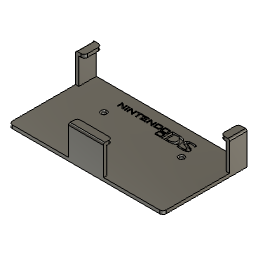
Nintendo DS Lite (Autodesk Fusion 360 design; units mm, degrees)
Autodesk Fusion 360 part; units mm, degrees
sketch "Sketch1" plane through (0, 0, 0) normal (0, 0, 1) x (1, 0, 0)
  line L0 (3, 0) -> (138, 0)
  line L1 (141, 3) -> (141, 77)
  line L2 (141, 77) -> (0, 77)
  line L3 (0, 77) -> (0, 3)
  line L4 (0, 77) -> (8, 77)
  line L5 (8, 77) -> (8, 61)
  line L6 (8, 61) -> (0, 61)
  line L7 (0, 61) -> (0, 77)
  line L8 (141, 77) -> (133, 77)
  line L9 (133, 77) -> (133, 64)
  line L10 (136, 61) -> (141, 61)
  line L11 (141, 61) -> (141, 77)
  line L12 (70.5, 77) -> (70.5, 0)
  line L13 (70.5, 0) -> (86.5, 0)
  line L14 (86.5, 0) -> (86.5, 5)
  line L15 (83.5, 8) -> (70.5, 8)
  line L16 (70.5, 8) -> (70.5, 0)
  line L17 (70.5, 0) -> (54.5, 0)
  line L18 (54.5, 0) -> (54.5, 5)
  line L19 (54.5, 8) -> (70.5, 8)
  line L20 (70.5, 8) -> (70.5, 0)
  line L21 (5, 61) -> (3, 61)
  line L22 (3, 61) -> (3, 77)
  line L23 (3, 77) -> (5, 77)
  line L24 (8, 74) -> (8, 64)
  line L25 (136, 77) -> (138, 77)
  line L26 (138, 77) -> (138, 61)
  line L27 (138, 61) -> (133, 61)
  line L28 (133, 61) -> (133, 74)
  line L29 (57.5, 8) -> (86.5, 8)
  line L30 (86.5, 8) -> (86.5, 3)
  line L31 (86.5, 3) -> (54.5, 3)
  line L32 (54.5, 3) -> (54.5, 8)
  arc A0 (8, 74) -> (5, 77) centre (5, 74) ccw
  arc A1 (136, 77) -> (133, 74) centre (136, 74) ccw
  arc A2 (133, 64) -> (136, 61) centre (136, 64) ccw
  arc A3 (5, 61) -> (8, 64) centre (5, 64) ccw
  arc A4 (57.5, 8) -> (54.5, 5) centre (57.5, 5) ccw
  arc A5 (86.5, 5) -> (83.5, 8) centre (83.5, 5) ccw
  arc A6 (0, 3) -> (3, 0) centre (3, 3) ccw
  arc A7 (138, 0) -> (141, 3) centre (138, 3) ccw
  point P0 (141, 0)
  dimension "d1" = 141
  dimension "d2" = 77
  dimension "d3" = 8
  dimension "d4" = 16
  dimension "d5" = 8
  dimension "d6" = 16
  dimension "d7" = 16
  dimension "d8" = 8
  dimension "d9" = 16
  dimension "d10" = 8
  dimension "d11" = 5
  dimension "d12" = 5
  dimension "d13" = 5
  dimension "d14" = 3
  dimension "d15" = 3
  dimension "d16" = 3
  dimension "d17" = 3
  constraint horizontal L0
  constraint vertical L1
  constraint horizontal L2
  constraint vertical L3
  constraint horizontal L4
  constraint vertical L5
  constraint horizontal L6
  constraint vertical L7
  constraint horizontal L8
  constraint vertical L9
  constraint horizontal L10
  constraint vertical L11
  constraint midpoint L2 L12.start
  constraint horizontal L13
  constraint vertical L14
  constraint horizontal L15
  constraint vertical L16
  constraint horizontal L17
  constraint vertical L18
  constraint horizontal L19
  constraint vertical L20
  constraint horizontal L21
  constraint vertical L22
  constraint horizontal L23
  constraint vertical L24
  constraint horizontal L25
  constraint vertical L26
  constraint horizontal L27
  constraint vertical L28
  constraint horizontal L29
  constraint vertical L30
  constraint horizontal L31
  constraint vertical L32
  constraint tangent L23 A0
  constraint tangent L24 A0
  constraint coincident L8.end L28
  constraint coincident L8.end L25
  constraint tangent L28 A1
  constraint tangent L25 A1
  constraint tangent L9 A2
  constraint tangent L10 A2
  constraint equal A1 A2
  constraint coincident L5.end L21
  constraint coincident L5.end L24
  constraint tangent L21 A3
  constraint tangent L24 A3
  constraint equal A1 A3
  constraint coincident L19.start L18
  constraint coincident L19.start L29
  constraint tangent L18 A4
  constraint tangent L29 A4
  constraint tangent L14 A5
  constraint tangent L15 A5
  constraint equal A4 A5
  constraint coincident L0 L12.end
  constraint coincident origin L0
  constraint coincident origin L3
  constraint tangent L0 A6
  constraint tangent L3 A6
  constraint coincident P0 L0
  constraint coincident P0 L1
  constraint tangent L0 A7
  constraint tangent L1 A7
  constraint equal A6 A7
  measures "d1" distance of origin P0
  measures "d2" distance of origin L2.end
  measures "d3" distance of L2.end L4.end
  measures "d4" distance of L2.end L6.end
  measures "d5" distance of L1.end L8.end
  measures "d6" distance of L1.end L10.end
  measures "d7" distance of L12.end L13.end
  measures "d8" distance of L12.end L15.end
  measures "d9" distance of L12.end L17.end
  measures "d10" distance of L12.end L15.end
  measures "d11" distance of L5.end L21.end
  measures "d12" distance of L8.end L25.end
  measures "d13" distance of L19.start L31.end
  measures "d14" radius of A0
  measures "d15" radius of A1
  measures "d16" radius of A4
  measures "d17" radius of A6
extrude "Extrude1" add sketch "Sketch1" along normal blind 30 contours L0 L12 L16 L17 L18 L20 L31 | L0 L12 L13 L14 L16 L20 L31 | L12 L16 L18 L19 L20 L29 L31 L32 A4 | L2 L3 L4 L6 L7 L22 | L12 L14 L15 L16 L20 L29 L30 L31 A5 | L2 L4 L5 L6 L21 L22 L23 L24 A0 A3 | L1 L2 L8 L10 L11 L26 | L2 L8 L9 L10 L25 L26 L27 L28 A1 A2 makes body 1 at (0, 71.6667, 10) makes body 2 at (141, 66.3333, 10) makes body 3 at (65.1667, 0, 10)
extrude "Extrude2" cut sketch "Sketch1" along normal blind 27 contours L12 L16 L18 L19 L20 L29 L31 L32 A4 | L12 L14 L15 L16 L20 L29 L30 L31 A5 | L2 L4 L5 L6 L21 L22 L23 L24 A0 A3 | L2 L8 L9 L10 L25 L26 L27 L28 A1 A2 bodies 1 2 3
extrude "Extrude3" add sketch "Sketch1" along normal blind 3 contours L0 L2 L3 L5 L6 L12 L18 L19 L21 L24 L29 L32 A6 | L12 L16 L18 L19 L20 L29 L31 L32 A4 | L0 L1 L2 L9 L10 L12 L14 L15 L27 L28 L29 L30 A7 | L12 L14 L15 L16 L20 L29 L30 L31 A5 | L19 L32 A4 | L2 L4 L5 L6 L21 L22 L23 L24 A0 A3 | L5 L6 A3 | L29 L30 A5 | L2 L4 L5 A0 | L2 L8 L9 A1 | L2 L8 L9 L10 L25 L26 L27 L28 A1 A2 | L27 L28 A2 bodies 1 2 3
fillet "Fillet1" radius 1.5 3 edges at (0, 69, 30) (70.5, 0, 30) (141, 69, 30) on bodies 1
sketch "Logo" plane through (0, 0, 3) normal (0, 0, 1) x (1, 0, 0)
  spline S0 degree 3 poles (75.8484, 66.8949) (75.8484, 67.0627) (75.8816, 67.0958) (76.0494, 67.0958) knots 0 0 0 0 1 1 1 1
  line L0 (76.0494, 67.0958) -> (79.7664, 67.0958)
  spline S1 degree 3 poles (79.7664, 67.0958) (79.9342, 67.0958) (79.9674, 67.0627) (79.9674, 66.8949) knots 2 2 2 2 3 3 3 3
  line L1 (79.9674, 66.8949) -> (79.9674, 64.2829)
  spline S2 degree 3 poles (79.9674, 64.2829) (79.9674, 64.1151) (79.9342, 64.082) (79.7664, 64.082) knots 4 4 4 4 5 5 5 5
  line L2 (79.7664, 64.082) -> (76.0494, 64.082)
  spline S3 degree 3 poles (76.0494, 64.082) (75.8816, 64.082) (75.8484, 64.1151) (75.8484, 64.2829) knots 6 6 6 6 7 7 7 7
  line L3 (75.8484, 64.2829) -> (75.8484, 66.8949)
  line L4 (75.0447, 66.9683) -> (75.0447, 64.2096)
  spline S4 degree 3 poles (75.0447, 64.2096) (75.0447, 63.6721) (75.4385, 63.2783) (75.976, 63.2783) knots 1 1 1 1 2 2 2 2
  line L5 (75.976, 63.2783) -> (79.8408, 63.2783)
  spline S5 degree 3 poles (79.8408, 63.2783) (80.3782, 63.2783) (80.7721, 63.6721) (80.7721, 64.2096) knots 3 3 3 3 4 4 4 4
  line L6 (80.7721, 64.2096) -> (80.7721, 66.9683)
  spline S6 degree 3 poles (80.7721, 66.9683) (80.7721, 67.5057) (80.3782, 67.8995) (79.8408, 67.8995) knots 5 5 5 5 6 6 6 6
  line L7 (79.8408, 67.8995) -> (75.976, 67.8995)
  spline S7 degree 3 poles (75.976, 67.8995) (75.4385, 67.8995) (75.0447, 67.5057) (75.0447, 66.9683) knots 7 7 7 7 8 8 8 8
  spline S8 degree 3 poles (75.8484, 61.6709) (75.8484, 61.8386) (75.8816, 61.8718) (76.0494, 61.8718) knots 0 0 0 0 1 1 1 1
  line L8 (76.0494, 61.8718) -> (79.7664, 61.8718)
  spline S9 degree 3 poles (79.7664, 61.8718) (79.9342, 61.8718) (79.9674, 61.8386) (79.9674, 61.6709) knots 2 2 2 2 3 3 3 3
  line L9 (79.9674, 61.6709) -> (79.9674, 59.0589)
  spline S10 degree 3 poles (79.9674, 59.0589) (79.9674, 58.8911) (79.9342, 58.8579) (79.7664, 58.8579) knots 4 4 4 4 5 5 5 5
  line L10 (79.7664, 58.8579) -> (76.0494, 58.8579)
  spline S11 degree 3 poles (76.0494, 58.8579) (75.8816, 58.8579) (75.8484, 58.8911) (75.8484, 59.0589) knots 6 6 6 6 7 7 7 7
  line L11 (75.8484, 59.0589) -> (75.8484, 61.6709)
  line L12 (75.0447, 61.7443) -> (75.0447, 58.9855)
  spline S12 degree 3 poles (75.0447, 58.9855) (75.0447, 58.4481) (75.4385, 58.0542) (75.976, 58.0542) knots 1 1 1 1 2 2 2 2
  line L13 (75.976, 58.0542) -> (79.8408, 58.0542)
  spline S13 degree 3 poles (79.8408, 58.0542) (80.3782, 58.0542) (80.7721, 58.4481) (80.7721, 58.9855) knots 3 3 3 3 4 4 4 4
  line L14 (80.7721, 58.9855) -> (80.7721, 61.7443)
  spline S14 degree 3 poles (80.7721, 61.7443) (80.7721, 62.2817) (80.3782, 62.6755) (79.8408, 62.6755) knots 5 5 5 5 6 6 6 6
  line L15 (79.8408, 62.6755) -> (75.976, 62.6755)
  spline S15 degree 3 poles (75.976, 62.6755) (75.4385, 62.6755) (75.0447, 62.2817) (75.0447, 61.7443) knots 7 7 7 7 8 8 8 8
  line L16 (40.8876, 67.8995) -> (40.0839, 67.8995)
  line L17 (40.1844, 63.2783) -> (40.8876, 63.2783)
  line L18 (35.8645, 63.2783) -> (36.6682, 63.2783)
  line L19 (35.8645, 67.8995) -> (35.8645, 63.2783)
  line L20 (40.0839, 64.4838) -> (36.6682, 67.8995)
  line L21 (40.8876, 63.2783) -> (40.8876, 67.8995)
  line L22 (36.6682, 66.7945) -> (40.1844, 63.2783)
  line L23 (36.6682, 63.2783) -> (36.6682, 66.7945)
  line L24 (36.6682, 67.8995) -> (35.8645, 67.8995)
  line L25 (40.0839, 67.8995) -> (40.0839, 64.4838)
  line L26 (49.5273, 67.8995) -> (48.7237, 67.8995)
  line L27 (45.3079, 66.7945) -> (48.8241, 63.2783)
  line L28 (44.5042, 63.2783) -> (45.3079, 63.2783)
  line L29 (49.5273, 63.2783) -> (49.5273, 67.8995)
  line L30 (44.5042, 67.8995) -> (44.5042, 63.2783)
  line L31 (45.3079, 63.2783) -> (45.3079, 66.7945)
  line L32 (48.7237, 64.4838) -> (45.3079, 67.8995)
  line L33 (48.7237, 67.8995) -> (48.7237, 64.4838)
  line L34 (45.3079, 67.8995) -> (44.5042, 67.8995)
  line L35 (48.8241, 63.2783) -> (49.5273, 63.2783)
  line L36 (63.1902, 63.2783) -> (63.1902, 66.7945)
  line L37 (66.6059, 64.4838) -> (63.1902, 67.8995)
  line L38 (63.1902, 67.8995) -> (62.3865, 67.8995)
  line L39 (66.6059, 67.8995) -> (66.6059, 64.4838)
  line L40 (63.1902, 66.7945) -> (66.7064, 63.2783)
  line L41 (62.3865, 63.2783) -> (63.1902, 63.2783)
  line L42 (62.3865, 67.8995) -> (62.3865, 63.2783)
  line L43 (67.4096, 67.8995) -> (66.6059, 67.8995)
  line L44 (67.4096, 63.2783) -> (67.4096, 67.8995)
  line L45 (66.7064, 63.2783) -> (67.4096, 63.2783)
  line L46 (42.2941, 67.8995) -> (43.0978, 67.8995)
  line L47 (43.0978, 67.8995) -> (43.0978, 63.2783)
  line L48 (42.2941, 63.2783) -> (42.2941, 67.8995)
  line L49 (43.0978, 63.2783) -> (42.2941, 63.2783)
  line L50 (53.5458, 63.2783) -> (53.5458, 67.0958)
  line L51 (50.532, 67.0958) -> (52.6417, 67.0958)
  line L52 (55.6555, 67.0958) -> (55.6555, 67.8995)
  line L53 (52.6417, 63.2783) -> (53.5458, 63.2783)
  line L54 (52.6417, 67.0958) -> (52.6417, 63.2783)
  line L55 (50.532, 67.8995) -> (50.532, 67.0958)
  line L56 (55.6555, 67.8995) -> (50.532, 67.8995)
  line L57 (53.5458, 67.0958) -> (55.6555, 67.0958)
  line L58 (61.0805, 67.8995) -> (56.5597, 67.8995)
  line L59 (57.4639, 64.082) -> (57.4639, 65.2875)
  line L60 (57.4639, 67.0958) -> (61.0805, 67.0958)
  line L61 (61.0805, 67.0958) -> (61.0805, 67.8995)
  line L62 (56.5597, 67.8995) -> (56.5597, 63.2783)
  line L63 (61.0805, 64.082) -> (57.4639, 64.082)
  line L64 (57.4639, 65.2875) -> (60.2768, 65.2875)
  line L65 (60.2768, 66.0912) -> (57.4639, 66.0912)
  line L66 (61.0805, 63.2783) -> (61.0805, 64.082)
  line L67 (57.4639, 66.0912) -> (57.4639, 67.0958)
  line L68 (56.5597, 63.2783) -> (61.0805, 63.2783)
  line L69 (60.2768, 65.2875) -> (60.2768, 66.0912)
  line L70 (69.6198, 67.0958) -> (72.3654, 67.0958)
  spline S16 degree 3 poles (72.3654, 67.0958) (72.9571, 67.0958) (73.4373, 66.4207) (73.4373, 65.5889) (73.4373, 64.7571) (72.9571, 64.082) (72.3654, 64.082) knots 1 1 1 1 2 2 2 3 3 3 3
  line L71 (72.3654, 64.082) -> (69.6198, 64.082)
  line L72 (69.6198, 64.082) -> (69.6198, 67.0958)
  line L73 (68.8161, 67.8995) -> (68.8161, 63.2783)
  line L74 (68.8161, 63.2783) -> (72.6336, 63.2783)
  spline S17 degree 3 poles (72.6336, 63.2783) (73.5217, 63.2783) (74.241, 64.313) (74.241, 65.5889) (74.241, 66.8648) (73.5217, 67.8995) (72.6336, 67.8995) knots 2 2 2 2 3 3 3 4 4 4 4
  line L75 (72.6336, 67.8995) -> (68.8161, 67.8995)
  line L76 (85.0909, 66.5935) -> (86.7666, 66.5935)
  spline S18 degree 3 poles (86.7666, 66.5935) (90.1994, 66.5935) (91.7214, 64.9741) (91.7214, 60.9797) (90.2346, 59.3603) (86.7666, 59.3603) knots 1 1 1 1 2 2 3 3 3 3
  line L77 (86.7666, 59.3603) -> (85.0909, 59.3603)
  line L78 (85.0909, 59.3603) -> (85.0909, 66.5935)
  line L79 (81.8762, 67.8995) -> (81.8762, 58.0542)
  line L80 (81.8762, 58.0542) -> (88.1048, 58.0542)
  spline S19 degree 3 poles (88.1048, 58.0542) (93.0274, 58.0542) (95.1372, 60.2583) (95.1372, 62.9769) (95.1372, 65.6954) (92.9772, 67.8995) (88.1048, 67.8995) knots 2 2 2 2 3 3 3 4 4 4 4
  line L81 (88.1048, 67.8995) -> (81.8762, 67.8995)
  spline S20 degree 3 poles (95.4516, 58.3606) (95.4516, 59.1342) (95.4295, 59.3984) (95.4295, 60.0364) knots 0 0 0 0 1 1 1 1
  spline S21 degree 3 poles (95.4295, 60.0364) (97.1193, 59.6175) (97.942, 59.4406) (99.1255, 59.3884) knots 1 1 1 1 2 2 2 2
  spline S22 degree 3 poles (99.1255, 59.3884) (99.5846, 59.3672) (100.4175, 59.3442) (100.8033, 59.4245) knots 2 2 2 2 3 3 3 3
  spline S23 degree 3 poles (100.8033, 59.4245) (101.188, 59.5049) (101.4402, 59.5501) (101.7134, 59.8234) knots 3 3 3 3 4 4 4 4
  spline S24 degree 3 poles (101.7134, 59.8234) (101.9866, 60.0967) (102.0077, 60.4221) (102.0077, 60.6281) (102.0077, 60.834) (101.8671, 60.9767) (101.7867, 61.0781) knots 4 4 4 4 5 5 5 6 6 6 6
  spline S25 degree 3 poles (101.7867, 61.0781) (101.6531, 61.2309) (101.409, 61.4007) (101.0564, 61.5886) knots 6 6 6 6 7 7 7 7
  spline S26 degree 3 poles (101.0564, 61.5886) (100.6325, 61.8327) (99.4058, 62.2476) (98.1027, 62.8072) knots 7 7 7 7 8 8 8 8
  ellipse E0 centre (110.6908, 60.1829) end of major axis (124.2883, 56.9811) minor radius 0.8448 (97.1986, 63.2391) -> (98.1027, 62.8072) ccw
  spline S27 degree 3 poles (97.1986, 63.2391) (96.646, 63.5285) (96.2413, 63.884) (95.9821, 64.1041) knots 9 9 9 9 10 10 10 10
  spline S28 degree 3 poles (95.9821, 64.1041) (95.7229, 64.3241) (95.6213, 64.5552) (95.5419, 64.7852) knots 10 10 10 10 11 11 11 11
  spline S29 degree 3 poles (95.5419, 64.7852) (95.4637, 65.0072) (95.4435, 65.1368) (95.4435, 65.39) (95.4435, 65.841) (95.5681, 66.3374) (95.9911, 66.7352) knots 11 11 11 11 12 12 12 13 13 13 13
  spline S30 degree 3 poles (95.9911, 66.7352) (96.415, 67.133) (97.0459, 67.4425) (97.8828, 67.6655) knots 13 13 13 13 14 14 14 14
  spline S31 degree 3 poles (97.8828, 67.6655) (98.7206, 67.8885) (99.7645, 68) (101.0132, 68) (101.7284, 68) (102.2439, 67.9568) (102.9461, 67.8543) knots 14 14 14 14 15 15 15 16 16 16 16
  spline S32 degree 3 poles (102.9461, 67.8543) (103.3218, 67.7991) (103.6634, 67.7036) (104.1908, 67.6403) knots 16 16 16 16 17 17 17 17
  spline S33 degree 3 poles (104.1908, 67.6403) (104.1908, 67.1139) (104.1857, 66.7603) (104.1857, 66.1123) knots 17 17 17 17 18 18 18 18
  spline S34 degree 3 poles (104.1857, 66.1123) (102.8024, 66.3886) (101.7435, 66.6508) (100.7711, 66.6508) (100.0759, 66.6508) (99.5173, 66.5604) (99.0924, 66.3805) knots 18 18 18 18 19 19 19 20 20 20 20
  spline S35 degree 3 poles (99.0924, 66.3805) (98.6684, 66.1997) (98.4253, 65.9978) (98.4253, 65.7788) (98.4253, 65.7135) (98.4253, 65.5919) (98.4334, 65.5025) knots 20 20 20 20 21 21 21 22 22 22 22
  spline S36 degree 3 poles (98.4334, 65.5025) (98.4394, 65.4241) (98.576, 65.2333) (98.6332, 65.168) knots 22 22 22 22 23 23 23 23
  ellipse E1 centre (103.246, 62.9964) end of major axis (107.9068, 60.7194) minor radius 0.3982 (98.6332, 65.168) -> (98.9608, 64.8997) ccw
  ellipse E2 centre (125.7124, 57.4495) end of major axis (152.6916, 49.714) minor radius 1.4569 (98.9608, 64.8997) -> (99.6911, 64.4878) ccw
  spline S37 degree 3 poles (99.6911, 64.4878) (100.0176, 64.3271) (101.0634, 64.0157) (101.3035, 63.9122) knots 25 25 25 25 26 26 26 26
  line L82 (101.3035, 63.9122) -> (102.712, 63.3868)
  spline S38 degree 3 poles (102.712, 63.3868) (103.0616, 63.213) (103.3971, 63.0914) (103.6805, 62.9226) knots 27 27 27 27 28 28 28 28
  spline S39 degree 3 poles (103.6805, 62.9226) (103.9637, 62.7528) (104.2099, 62.5881) (104.4199, 62.4263) knots 28 28 28 28 29 29 29 29
  spline S40 degree 3 poles (104.4199, 62.4263) (104.6298, 62.2656) (104.7393, 62.132) (104.8629, 61.9813) knots 29 29 29 29 30 30 30 30
  spline S41 degree 3 poles (104.8629, 61.9813) (104.9854, 61.8296) (105.0749, 61.5785) (105.1351, 61.4217) knots 30 30 30 30 31 31 31 31
  spline S42 degree 3 poles (105.1351, 61.4217) (105.1954, 61.265) (105.2275, 60.8963) (105.2275, 60.7265) (105.2275, 60.3207) (105.0969, 59.936) (104.8076, 59.5501) knots 31 31 31 31 32 32 32 33 33 33 33
  spline S43 degree 3 poles (104.8076, 59.5501) (104.5223, 59.1704) (104.039, 58.7906) (103.4533, 58.5606) knots 33 33 33 33 34 34 34 34
  spline S44 degree 3 poles (103.4533, 58.5606) (102.8687, 58.3305) (102.2077, 58.1859) (101.5226, 58.0984) knots 34 34 34 34 35 35 35 35
  spline S45 degree 3 poles (101.5226, 58.0984) (100.8384, 58.011) (100.2878, 58) (99.5274, 58) (99.017, 58) (98.2906, 58.0794) (97.6416, 58.1286) (96.9927, 58.1779) (96.641, 58.2049) (95.4516, 58.3606) knots 35 35 35 35 36 36 36 37 37 37 38 38 38 38
extrude "Extrude4" cut sketch "Logo" against normal blind 2 bodies 1
hole "Hole1" at (35, 52, 3) direction (0, 0, -1) diameter 3.5 depth 3 tip angle 118 countersink diameter 5.5 countersink angle 90 bodies 1
hole "Hole2" at (106, 52, 3) direction (0, 0, -1) diameter 3.5 depth 3 tip angle 118 countersink diameter 5.5 countersink angle 90 bodies 1
